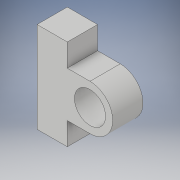
# Autodesk Inventor part: Achsenhalterung
Saved by Autodesk Inventor 2018 (Build 220112000, 112)
## iProperties
Created: 2018-01-20
Part Number: Achsenhalterung
Material: Generisch
Document SubType Name: Modeling
Designer: Administrator
Density: 1 g/cm^3
Appearance: Vorgabe
Author: Administrator
Autodesk Inventor part; units mm, degrees
ref_plane "YZ Plane" through (0, 0, 0) normal (1, 0, 0) x (0, 1, 0)
ref_plane "XZ Plane" through (0, 0, 0) normal (0, 1, 0) x (-1, 0, 0)
ref_plane "XY Plane" through (0, 0, 0) normal (0, 0, 1) x (1, 0, 0)
sketch "Skizze1" plane through (0, 0, 0) normal (0, 1, 0) x (-1, 0, 0)
  line L0 (-1.8, 15) -> (8.2, 15)
  line L1 (8.2, 15) -> (8.2, -15)
  line L2 (8.2, -15) -> (-1.8, -15)
  line L3 (16.5068, 0) -> (-47.7946, 0) construction
  arc A0 (-9.3, 7.5) -> (-9.3, -7.5) centre (-9.3, 0) ccw
  circle A1 centre (-9.3, 0) radius 5.15
  line L4 (-1.8, -15) -> (-1.8, -7.5)
  line L5 (-1.8, 7.5) -> (-1.8, 15)
  line L6 (-9.3, 7.5) -> (-1.8, 7.5)
  line L7 (-9.3, -7.5) -> (-1.8, -7.5)
  point P0 (0, 0)
  dimension "d0" = 30
  dimension "d1" = 15
  dimension "d2" = 10.3
  dimension "d3" = 15
  dimension "d7" = 10
  dimension "d8" = 17.5
  dimension "d14" = 7.5
  dimension "d15" = 7.5
  dimension "d16" = 1.8
  dimension "d17" = 1.8
  constraints: 16 end point, 5 perpendicular, 4 point on circle, 4 point on line, 3 horizontal, 2 centre point, 1 coincident
  measures "d0" distance of L0.end L1.end
  measures "d1" distance between parallel lines of L2 L3
  measures "d2" diameter of A1
  measures "d3" diameter of A0
  measures "d7" distance between parallel lines of L5 L1
  measures "d8" distance from line of L1 A1.centre
  measures "d14" distance from line of L6 L0.start
  measures "d15" distance of L2.end L4.end
  measures "d16" distance from line of point (0, 0) L5
  measures "d17" horizontal distance of point (0, 0) L4.end
extrude "Extrusion1" add sketch "Skizze1" along normal blind 10
